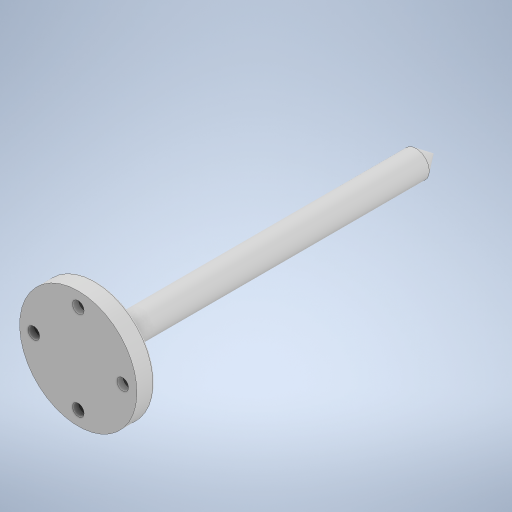
# Autodesk Inventor part: Drzak_kamera
Saved by Autodesk Inventor 2023 (Build 270158000, 158)
## iProperties
Created: 2025-01-03
Part Number: Drzak_kamera
Material: Všeobecné
Document SubType Name: Modeling
Designer: LISNÍK P.
Density: 1 g/cm^3
Appearance: Výchozí
Author: LISNÍK P.
Autodesk Inventor part; units mm, degrees
ref_plane "YZ Plane" through (0, 0, 0) normal (1, 0, 0) x (0, 1, 0)
ref_plane "XZ Plane" through (0, 0, 0) normal (0, 1, 0) x (-1, 0, 0)
ref_plane "XY Plane" through (0, 0, 0) normal (0, 0, 1) x (1, 0, 0)
sketch "Náčrt11" plane through (0, 0, 0) normal (1, 0, 0) x (0, 1, 0)
  line L0 (-6.6, 0) -> (39.6, 0) projected
  line L1 (0, -240) -> (0, 40) projected
  line L2 (0, 0) -> (33, 0)
  line L3 (33, 0) -> (33, -10)
  line L4 (33, -10) -> (0, -10)
  line L5 (0, -10) -> (0, 0)
  line L6 (0, -10) -> (7.5, -10)
  line L7 (7.5, -10) -> (7.5, -200)
  line L8 (7.5, -200) -> (0, -200)
  line L9 (0, -200) -> (0, -10)
  point P0 (33, 0)
  point P1 (0, -200)
  dimension "d109" = 33
  dimension "d110" = 10
  dimension "d111" = 7.5
  dimension "d112" = 190
  constraints: 16 end point, 4 parallel, 2 horizontal, 2 perpendicular
  measures "d109" distance of L3.end L4.end
  measures "d110" distance of L2.end L3.end
  measures "d111" distance of L7.end L8.end
  measures "d112" distance of L6.end L7.end
revolve "Rotace2" add sketch "Náčrt11" angle 360 about axis through (0, 0, -10) along (0, 0, 1)
sketch "Náčrt12" plane through (0, 0, -10) normal (0, 0, -1) x (-1, 0, 0)
  line L0 (46.2, 0) -> (-46.2, 0) projected
  line L1 (0, -46.2) -> (0, 46.2) projected
  circle A0 centre (0, 0) radius 25 construction
  point P0 (0, 25)
  point P1 (-25, 0)
  point P2 (25, 0)
  point P3 (0, -25)
  dimension "d114" = 50
  constraints: 4 point on circle, 4 point on line, 1 centre point, 1 coincident
  measures "d114" diameter of A0
hole "Díra4" at (0, 25, -10) at (25, 0, -10) at (-25, 0, -10) at (0, -25, -10) direction (0, 0, 1) diameter 6.6 end through all counterbore diameter 11.4 counterbore depth 6.5 clearance for "Šroub s hlavou s vnitřním vybráním ISO 4762" size "M6" standard "ISO"
chamfer "Zkosení4" distance 10 distance2 7.5 1 edges at (0, -7.5, -200) measured on face at (0.6035, 7.4757, -136.6667)
fillet "Zaoblení12" radius 1 1 edges at (0, -33, -10)
fillet "Zaoblení13" radius 10 1 edges at (0, -7.5, -10)
